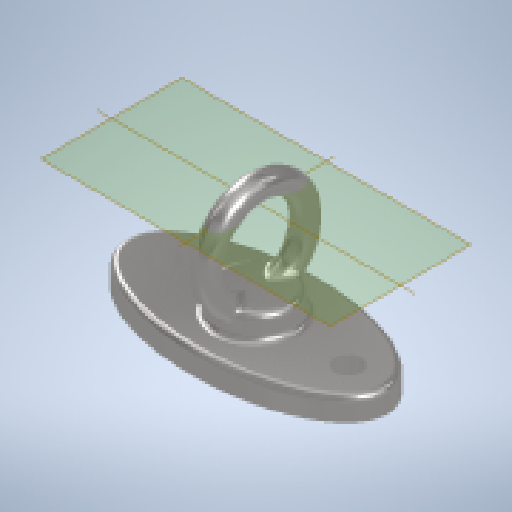
# Autodesk Inventor part: hook
Saved by Autodesk Inventor 2024 (Build 280153000, 153)
## iProperties
Created: 2023-05-24
Part Number: hook
Material: Steel, Galvanized
Document SubType Name: Modeling
Designer: Patrick
Density: 7.85 g/cm^3
Appearance: Galvanized
Author: Patrick
Autodesk Inventor part; units mm, degrees
ref_plane "XZ Plane" through (0, 0, 0) normal (0, 1, 0) x (-1, 0, 0)
sketch "Sketch1" plane through (0, 0, 0) normal (0, 1, 0) x (-1, 0, 0)
  ellipse E0 centre (0, 0) end of major axis (-40, 0) minor radius 19.5
  line L0 (-56, 0) -> (56, 0) construction
  line L1 (0, -27.3) -> (0, 27.3) construction
  point P0 (40, 0)
  point P1 (-40, 0)
  point P2 (0, -19.5)
  point P3 (0, 19.5)
  dimension "d1" = 80
  dimension "d2" = 39
  constraints: 4 point on line, 1 coincident, 6 other
  measures "d1" distance of point (-40, 0) point (40, 0)
  measures "d2" distance of point (0, 19.5) point (0, -19.5)
extrude "Extrusion1" add sketch "Sketch1" along normal blind 7
sketch "Sketch2" plane through (0, 7, 0) normal (0, 1, 0) x (1, 0, 0)
  circle A0 centre (0, 0) radius 11
  dimension "d5" = 22
  constraints: 1 centre point, 1 coincident
  measures "d5" diameter of A0
extrude "Extrusion2" add sketch "Sketch2" along normal blind 7
fillet "Fillet1" radius 2 3 edges at (-11, 14, 0) (-40, 7, 0) (-11, 7, 0)
sketch "Sketch3" plane through (0, 0, 0) normal (0, 0, 1) x (1, 0, 0)
  line L0 (0, 28.8) -> (0, -4.8) construction
  circle A0 centre (0, 10) radius 3.5
  line L1 (11, 14) -> (-11, 14) construction
  line L2 (-39.2168, 25) -> (38.0745, 25)
  point P0 (0, 0)
  point P1 (0, 13.5)
  dimension "d8" = 7
  dimension "d9" = 4
  dimension "d11" = 23
  constraints: 2 end point, 2 point on line, 1 horizontal, 1 vertical alignment, 2 other
  measures "d9" distance from line of L1 point (0, 10)
  measures "d11" diameter of point (0, 13.5) L2
revolve "Revolution1" add sketch "Sketch3" angle 360 about axis through (-39.2168, 25, 0) along (1, 0, 0)
fillet "Fillet2" radius 2 10 edges at (-3.4923, 13.3793, -9.8474) (-0.0042, 10.1255, -11) (3.4381, 13.8775, -9.0586) (3.3745, 12.8316, -10.2792) (0.0017, 14, -3.3541) (-0.0042, 10.1255, 11) (-3.4923, 13.3793, 9.8474) (0.0017, 14, 3.3541) (3.3744, 12.8315, 10.2792) (3.4381, 13.8775, 9.0586)
sketch "Sketch4" plane through (0, 7, 0) normal (0, 1, 0) x (1, 0, 0)
  line L0 (-28, 0) -> (28, 0) construction
  point P0 (0, 0)
  point P1 (0, 0)
  dimension "d16" = 56
  constraints: 2 end point, 1 coincident, 1 horizontal, 1 midpoint
  measures "d16" distance of L0.start L0.end
hole "Hole1" at (-28, 7, 0) at (28, 7, 0) direction (0, -1, 0) diameter 8 end through all
ref_plane "Work Plane3" through (0, 36, 0) normal (0, -1, 0) x (1, 0, 0)
body "Solid1"
